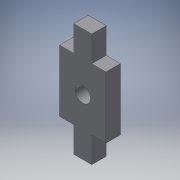
# Autodesk Inventor part: Part19
Saved by Autodesk Inventor 2019.2 (Build 232265000, 265)
## iProperties
Created: 2019-04-03
Part Number: Part19
Material: Generic
Document SubType Name: Modeling
Designer: richard.girt
Mass: 0.380608 g
Surface Area: 4.71852 cm^2
Volume: 0.380608 cm^3
Density: 1 g/cm^3
Appearance: Default
Author: richard.girt
Autodesk Inventor part; units mm, degrees
note: some values were not read from the file. Chosen so that the rebuilt part matches the saved one: sketch regions of "Extrusion1".
ref_plane "YZ Plane" through (0, 0, 0) normal (1, 0, 0) x (0, 1, 0)
ref_plane "XZ Plane" through (0, 0, 0) normal (0, 1, 0) x (-1, 0, 0)
ref_plane "XY Plane" through (0, 0, 0) normal (0, 0, 1) x (1, 0, 0)
sketch "Sketch1" plane through (0, 0, 0) normal (0, 0, 1) x (1, 0, 0)
  line L0 (-4.5, -6) -> (4.5, -6)
  line L1 (4.5, -6) -> (4.5, 6)
  line L2 (4.5, 6) -> (-4.5, 6)
  line L3 (-4.5, 6) -> (-4.5, -6)
  line L4 (-1.75, 11) -> (1.75, 11)
  line L5 (1.75, -11) -> (-1.75, -11)
  circle A0 centre (0, 0) radius 1.5
  line L6 (1.75, 11) -> (1.75, 6)
  line L7 (1.75, -6) -> (1.75, -11)
  line L8 (-1.75, -11) -> (-1.75, -6)
  line L9 (-1.75, 6) -> (-1.75, 11)
  dimension "d0" = 3
  dimension "d1" = 12
  dimension "d2" = 9
  dimension "d3" = 3.5
  dimension "d4" = 11
  dimension "d5" = 22
  dimension "d6" = 1.75
  dimension "d7" = 4.5
  constraints: 20 end point, 5 vertical, 4 point on line, 3 equal length, 2 horizontal, 1 centre point, 1 vertical alignment
  measures "d0" diameter of A0
  measures "d1" distance of L0.end L1.end
  measures "d2" distance of L0.start L0.end
  measures "d3" distance between parallel lines of L8 L7
  measures "d4" distance from line of point (0, 0) L5
  measures "d5" distance between parallel lines of L4 L5
  measures "d6" distance from line of L8 point (0, 0)
  measures "d7" distance from line of L3 point (0, 0)
extrude "Extrusion1" add sketch "Sketch1" along normal mid plane 2.8
equation "\"d4\" = 0.5 * d5"
equation "\"d6\" = 0.5 * d3"
equation "\"d7\" = 0.5 * d2"
body "Solid1"
